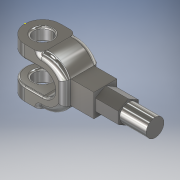
# Autodesk Inventor part: Double Eye End
Saved by Autodesk Inventor 2018 (Build 220112000, 112)
## iProperties
Created: 2019-09-01
Part Number: Double Eye End
Material: Generic
Document SubType Name: Modeling
Designer: Sameer
Density: 1 g/cm^3
Appearance: Chrome - Polished
Author: Sameer
Autodesk Inventor part; units mm, degrees
ref_plane "YZ Plane" through (0, 0, 0) normal (1, 0, 0) x (0, 1, 0)
ref_plane "XZ Plane" through (0, 0, 0) normal (0, 1, 0) x (-1, 0, 0)
ref_plane "XY Plane" through (0, 0, 0) normal (0, 0, 1) x (1, 0, 0)
sketch "Sketch1" plane through (0, 0, 0) normal (0, 0, 1) x (1, 0, 0)
  line L0 (0, 13) -> (0, 28)
  line L1 (0, 28) -> (40, 28)
  line L2 (40, -28) -> (0, -28)
  line L3 (0, -28) -> (0, -13)
  line L4 (0, -13) -> (40, -13)
  line L5 (0, 13) -> (40, 13)
  arc A0 (40, -13) -> (40, 13) centre (40, 0) ccw
  line L6 (64.8682, 13) -> (90.8682, 13)
  line L7 (90.8682, 13) -> (90.8682, -13)
  line L8 (90.8682, -13) -> (64.8682, -13)
  arc A1 (38.1492, -28) -> (64.8682, -13) centre (40, 0) ccw
  arc A2 (64.8682, 13) -> (38.1492, 28) centre (40, 0) ccw
  point P0 (0, 0)
  dimension "d0" = 15
  dimension "d1" = 40
  dimension "d2" = 56
  dimension "d3" = 15
  dimension "d5" = 26
  dimension "d6" = 90.8682
  constraints: 18 end point, 6 point on circle, 4 point on line, 3 centre point, 3 perpendicular, 1 coincident, 1 horizontal, 1 vertical
  measures "d0" distance of L0.start L0.end
  measures "d1" distance of L0.end L1.end
  measures "d2" distance of L1.end L2.start
  measures "d3" distance of L2.end L3.end
  measures "d5" distance of L6.end L7.end
  measures "d6" distance between parallel lines of L7 L0
extrude "Extrusion1" add sketch "Sketch1" along normal mid plane 40
sketch "Sketch2" plane through (0, 28, 20) normal (0, 1, 0) x (1, 0, 0)
  point P0 (0, 20)
sketch "Sketch3" plane through (0, 28, 20) normal (0, 1, 0) x (1, 0, 0)
  arc A0 (35.1987, 33) -> (35.1987, 7) centre (20, 20) ccw
  circle A1 centre (20, 20) radius 10
  line L0 (40, 20) -> (90.8682, 20)
  line L1 (35.1987, 7) -> (90.8682, 7)
  line L2 (35.1987, 33) -> (90.8682, 33)
  line L3 (90.8682, 0) -> (90.8682, 40) projected
  line L4 (90.8682, 7) -> (90.8682, 33)
  point P0 (0, 20)
  dimension "d10" = 20
  dimension "d11" = 13
  dimension "d12" = 13
  constraints: 8 end point, 3 point on circle, 2 centre point, 2 parallel, 2 point on line, 1 coincident, 1 horizontal, 1 midpoint
  measures "d10" diameter of A1
  measures "d11" distance between parallel lines of L0 L1
  measures "d12" distance between parallel lines of L0 L2
extrude "Extrusion2" cut sketch "Sketch3" against normal through all contours A1
fillet "Fillet1" radius 20 4 edges at (0, 20.5, 20) (0, 20.5, -20) (0, -20.5, 20) (0, -20.5, -20)
sketch "Sketch4" plane through (64.8682, 13, 20) normal (0, 1, 0) x (1, 0, 0)
  point P0 (-64.8682, 20)
sketch "Sketch5" plane through (90.8682, -13, 20) normal (1, 0, 0) x (0, 0, -1)
  line L0 (0, 0) -> (40, 0)
  line L1 (40, 0) -> (40, 26)
  line L2 (40, 26) -> (0, 26)
  line L3 (0, 26) -> (0, 0)
  line L4 (0, 0) -> (40, 26) construction
  line L5 (40, 0) -> (0, 26) construction
  point P0 (20, 13)
  dimension "d16" = 40
  dimension "d17" = 26
  constraints: 12 end point, 2 midpoint, 2 parallel, 1 horizontal, 1 perpendicular
  measures "d16" distance of L2.end L1.end
  measures "d17" distance of L0.end L1.end
extrude "Extrusion3" cut sketch "Sketch5" against normal blind 26
sketch "Sketch6" plane through (64.8682, -13, 20) normal (1, 0, 0) x (0, 0, -1)
  line L0 (40, 26) -> (0, 26) projected
  line L1 (7, 0) -> (33, 0)
  line L2 (33, 0) -> (33, 26)
  line L3 (33, 26) -> (7, 26)
  line L4 (7, 26) -> (7, 0)
  line L5 (7, 0) -> (33, 26) construction
  line L6 (33, 0) -> (7, 26) construction
  point P0 (20, 13)
  dimension "d20" = 26
  constraints: 12 end point, 2 midpoint, 2 parallel, 1 horizontal, 1 perpendicular, 1 point on line
  measures "d20" distance of L3.end L2.end
extrude "Extrusion4" add sketch "Sketch6" along normal blind 26
fillet "Fillet2" radius 7 6 edges at (64.8682, 0, -20) (53.7368, 24.4689, -20) (53.7368, -24.4689, -20) (53.7368, -24.4689, 20) (64.8682, 0, 20) (53.7368, 24.4689, 20)
sketch "Sketch7" plane through (90.8682, -13, 20) normal (1, 0, 0) x (0, 0, -1)
  line L0 (0, 0) -> (40, 0) projected
  line L1 (20, 0) -> (8.7417, 6.5)
  line L2 (8.7417, 6.5) -> (8.7417, 19.5)
  line L3 (8.7417, 19.5) -> (20, 26)
  line L4 (20, 26) -> (31.2583, 19.5)
  line L5 (31.2583, 19.5) -> (31.2583, 6.5)
  line L6 (31.2583, 6.5) -> (20, 0)
  point P0 (20, 13)
  point P1 (20, 13)
  constraints: 12 end point, 1 coincident, 1 midpoint, 13 other
extrude "Extrusion5" add sketch "Sketch7" along normal blind 26
sketch "Sketch8" plane through (116.8682, -13, 20) normal (1, 0, 0) x (0, 0, -1)
  circle A0 centre (20, 13) radius 10
  dimension "d26" = 20
  constraints: 1 centre point, 1 coincident
  measures "d26" diameter of A0
extrude "Extrusion6" add sketch "Sketch8" along normal blind 30
fillet "Fillet3" radius 2 15 edges at (10, -28, 0) (29.9999, 13, 20) (53, 0, 20) (29.9999, -13, 20) (5.8578, -13, -14.1422) (0, -13, 0) (5.8578, -13, 14.1422) (29.9999, -13, -20) (53, 0, -20) (29.9999, 13, -20) (0, 13, 0) (5.8578, 13, -14.1422) (5.8578, 13, 14.1422) (10, 13, 0) (10, -13, 0)
fillet "Fillet4" radius 2 1 edges at (10, 28, 0)
body "Solid1"
